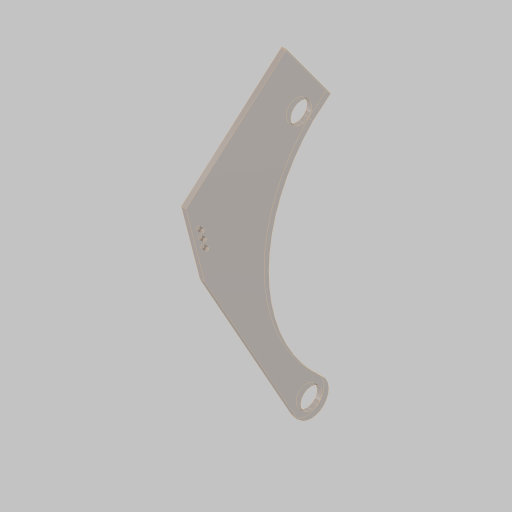
# Autodesk Inventor part: GP4-001
Saved by Autodesk Inventor 2023.5 (Build 275446000, 446)
## iProperties
Created: 2025-01-28
Part Number: GP4-001
Material: Polycarbonate, Smoke
Document SubType Name: Modeling
Designer: slick
Density: 1.2 g/cm^3
Appearance: Polycarbonate - Smoked
Author: slick
Autodesk Inventor part; units mm, degrees
ref_plane "YZ Plane" through (0, 0, 0) normal (1, 0, 0) x (0, 1, 0)
ref_plane "XZ Plane" through (0, 0, 0) normal (0, 1, 0) x (-1, 0, 0)
ref_plane "XY Plane" through (0, 0, 0) normal (0, 0, 1) x (1, 0, 0)
sketch "Sketch1" plane through (0, 0, 0) normal (1, 0, 0) x (0, 1, 0)
  circle A0 centre (0, 0) radius 203.2 construction
  circle A1 centre (165.1, 167.1631) radius 38.1 construction
  circle A2 centre (165.1, 167.1631) radius 31.75 construction
  circle A3 centre (-177.8, 153.586) radius 38.1 construction
  circle A4 centre (-177.8, 153.586) radius 31.75 construction
  circle A5 centre (279.4, 30.6697) radius 38.1 construction
  circle A6 centre (279.4, 30.6697) radius 31.75 construction
  line L0 (371.6722, 159.6086) -> (293.9242, 243.3925) construction
  line L1 (293.9242, 243.3925) -> (72.8278, 38.2242) construction
  line L2 (72.8278, 38.2242) -> (150.5758, -45.5597) construction
  line L3 (150.5758, -45.5597) -> (371.6722, 159.6086) construction
  line L4 (371.6722, 159.6086) -> (72.8278, 38.2242) construction
  line L5 (293.9242, 243.3925) -> (150.5758, -45.5597) construction
  line L6 (165.1, 167.1631) -> (279.4, 30.6697) construction
  point P0 (222.25, 98.9164)
  dimension "d0" = 406.4
  dimension "d1" = 76.2
  dimension "d2" = 6.35
  dimension "d4" = 114.3
  dimension "d5" = 301.625
  dimension "d6" = 177.8
  dimension "d51" = 165.1
  dimension "d52" = 279.4
  dimension "d53" = 30.6697
  constraints: 14 end point, 7 centre point, 4 equal radius, 4 tangent, 3 midpoint, 2 coincident, 2 parallel, 1 perpendicular
  measures "d0" diameter of A0
  measures "d1" diameter of A1
  measures "d2" radial gap between concentric circles of A1 A2
  measures "d4" distance of L2.end L1.end
  measures "d5" distance of L1.end L0.end
  measures "d6" horizontal distance of A3.centre point (0, 0)
  measures "d51" horizontal distance of point (0, 0) L6.start
  measures "d52" horizontal distance of point (0, 0) L6.end
  measures "d53" vertical distance of point (0, 0) L6.end
sketch "Sketch4" plane through (0, 0, 0) normal (1, 0, 0) x (0, 1, 0)
  circle A0 centre (0, 0) radius 203.2 construction
  circle A1 centre (165.1, 167.1631) radius 38.1 construction
  circle A2 centre (165.1, 167.1631) radius 31.75 construction
  circle A3 centre (-177.8, 153.586) radius 38.1 construction
  circle A4 centre (-177.8, 153.586) radius 31.75 construction
  circle A5 centre (279.4, 30.6697) radius 38.1 construction
  circle A6 centre (279.4, 30.6697) radius 31.75 construction
  line L0 (371.6722, 159.6086) -> (293.9242, 243.3925) construction
  line L1 (293.9242, 243.3925) -> (72.8278, 38.2242) construction
  line L2 (72.8278, 38.2242) -> (150.5758, -45.5597) construction
  line L3 (150.5758, -45.5597) -> (371.6722, 159.6086) construction
  line L4 (371.6722, 159.6086) -> (72.8278, 38.2242) construction
  line L5 (293.9242, 243.3925) -> (150.5758, -45.5597) construction
  line L6 (165.1, 167.1631) -> (279.4, 30.6697) construction
  circle A7 centre (-177.8, 153.586) radius 14.2875
  circle A8 centre (165.1, 167.1631) radius 14.2875
  circle A9 centre (279.4, 30.6697) radius 14.2875
  circle A10 centre (165.1, 167.1631) radius 23.8125 construction
  circle A11 centre (279.4, 30.6697) radius 23.8125 construction
  circle A12 centre (-177.8, 153.586) radius 23.8125 construction
  line L7 (261.1433, 15.3815) -> (146.8433, 151.8749)
  line L8 (309.92, 115.3835) -> (248.7672, 188.4102)
  line L9 (309.92, 115.3835) -> (303.1398, 28.8105)
  line L10 (248.7672, 188.4102) -> (130.1238, 323.85)
  line L11 (130.1238, 323.85) -> (31.75, 298.45)
  line L12 (31.75, 298.45) -> (-189.4509, 174.3536)
  arc A13 (148.3669, 150.2209) -> (-159.7797, 138.0199) centre (0, 0) ccw
  arc A14 (148.3669, 150.2209) -> (146.8433, 151.8749) centre (165.1, 167.1631) ccw
  arc A15 (256.4562, 24.2964) -> (303.1398, 28.8105) centre (279.4, 30.6697) ccw
  line L13 (332.7982, 201.5005) -> (111.7018, -3.6678) construction
  arc A16 (-189.4509, 174.3536) -> (-159.7797, 138.0199) centre (-177.8, 153.586) ccw
  point P0 (222.25, 98.9164)
  point P1 (279.3436, 151.8969)
  point P2 (261.1433, 15.3815)
  point P3 (147.5854, 150.9888)
  dimension "d27" = 28.575
  dimension "d29" = 9.525
  dimension "d31" = 101.6
  dimension "d33" = 101.6
  dimension "d35" = 95.25
  dimension "d58" = 298.45
  dimension "d59" = 323.85
  dimension "d60" = 31.75
  constraints: 15 end point, 15 point on circle, 10 centre point, 7 coincident, 5 equal radius, 5 tangent, 3 midpoint, 1 parallel, 1 point on line
  measures "d27" diameter of A7
  measures "d29" radial gap between concentric circles of A9 A11
  measures "d31" distance between parallel lines of L7 L8
  measures "d33" distance of L10.end L11.end
  measures "d35" distance of L8.start L8.end
  measures "d58" vertical distance of point (0, 0) L11.end
  measures "d59" vertical distance of point (0, 0) L10.end
  measures "d60" horizontal distance of point (0, 0) L11.end
extrude "Extrusion2" add sketch "Sketch4" along normal blind 6.35 contours L7 A14 A13 | L7 A13 A16 L12 L11 L10 L8 L9 A15
sketch "Sketch5" plane through (6.35, 0, 0) normal (1, 0, 0) x (0, 0, -1)
  line L0 (-323.85, 130.1238) -> (-298.45, 31.75) projected
  line L1 (-301.2085, 93.2336) -> (-294.8585, 68.6402) construction
  point P0 (0, 0)
  point P1 (-298.0335, 80.9369)
  point P2 (-311.15, 80.9369)
  point P3 (-298.0335, 80.9369)
  point P4 (-311.15, 80.9369)
  dimension "d39" = 12.7
  dimension "d57" = 25.4
  constraints: 3 midpoint, 2 end point, 1 coincident, 1 horizontal alignment, 1 parallel
  measures "d39" distance from line of L0 L1.start
  measures "d57" distance of L1.start L1.end
hole "Hole2" at (6.35, 93.2336, 301.2085) at (6.35, 80.9369, 298.0335) at (6.35, 68.6402, 294.8585) direction (-1, 0, 0) diameter 5.1054 end through all clearance for "Flat Head Machine Screw (82)" size "#10" standard "Ansi Unified Screw Threads"
sketch "Sketch6" plane through (6.35, 0, 0) normal (1, 0, 0) x (0, 0, -1)
  line L0 (-187.1778, 249.7992) -> (-127.0195, 167.6573)
  circle A0 centre (-298.0335, 80.9369) radius 2.5527 projected
  circle A1 centre (-301.2085, 93.2336) radius 2.5527 projected
  circle A2 centre (-294.8585, 68.6402) radius 2.5527 projected
  arc A3 (-15.3815, 261.1433) -> (-28.8105, 303.1398) centre (-30.6697, 279.4) ccw projected
  line L1 (-28.8105, 303.1398) -> (-115.3835, 309.92) projected
  line L2 (-115.3835, 309.92) -> (-188.4102, 248.7672) projected
  line L3 (-188.4102, 248.7672) -> (-323.85, 130.1238) projected
  line L4 (-323.85, 130.1238) -> (-298.45, 31.75) projected
  line L5 (-298.45, 31.75) -> (-174.3536, -189.4509) projected
  arc A4 (-174.3536, -189.4509) -> (-138.0199, -159.7797) centre (-153.586, -177.8) ccw projected
  arc A5 (-150.9888, 147.5854) -> (-138.0199, -159.7797) centre (0, 0) ccw projected
  line L6 (-150.9888, 147.5854) -> (-15.3815, 261.1433) projected
  circle A6 centre (-30.6697, 279.4) radius 14.2875 projected
  circle A7 centre (-167.1631, 165.1) radius 14.2875 projected
  circle A8 centre (-153.586, -177.8) radius 14.2875 projected
  dimension "d61" = 180.975
  dimension "d62" = 85
  constraints: 2 end point, 2 point on line
  measures "d61" distance from line of L3.end L0
  measures "d62" angle of L3 L0
extrude "Extrusion3" cut sketch "Sketch6" against normal blind 25.4 contours L2 L1 A3 L6 L0
body "Solid2"
